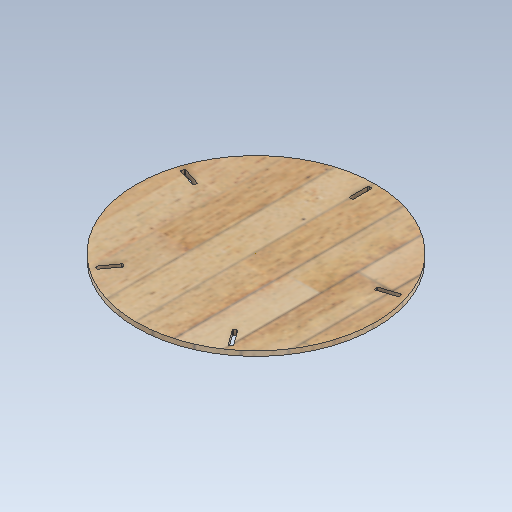
# Autodesk Inventor part: fINAL Roof - G
Saved by Autodesk Inventor 2020 (Build 240168000, 168)
## iProperties
Created: 2020-03-07
Part Number: fINAL Roof - G
Material: Wood (Maple)
Document SubType Name: Sheet Metal
Designer: Daniel Wikman
Density: 0.67 g/cm^3
Sheet Metal Rule: Default_mm
Appearance: Natural Maple - Glossy Dark Tint
Author: Daniel Wikman
Autodesk Inventor part; units mm, degrees
ref_plane "YZ Plane" through (0, 0, 0) normal (1, 0, 0) x (0, 1, 0)
ref_plane "XZ Plane" through (0, 0, 0) normal (0, 1, 0) x (-1, 0, 0)
ref_plane "XY Plane" through (0, 0, 0) normal (0, 0, 1) x (1, 0, 0)
sketch "Sketch1" plane through (0, 0, 0) normal (0, 1, 0) x (-1, 0, 0)
  circle A0 centre (0, 0) radius 200
  dimension "d0" = 400
  constraints: 1 centre point, 1 coincident
  measures "d0" diameter of A0
extrude "Extrusion1" add sketch "Sketch1" along normal blind 8
sketch "Sketch2" plane through (0, 8, 0) normal (0, 1, 0) x (1, 0, 0)
  line L0 (-1.9167, 191.4) -> (1.9167, 191.4)
  line L1 (3.25, 190.0667) -> (3.25, 160.0667)
  line L2 (1.9167, 158.7333) -> (-1.9167, 158.7333)
  line L3 (-3.25, 160.0667) -> (-3.25, 190.0667)
  circle A0 centre (0, 0) radius 200 projected
  arc A1 (-1.9167, 191.4) -> (-3.25, 190.0667) centre (-1.9167, 190.0667) ccw
  arc A2 (3.25, 190.0667) -> (1.9167, 191.4) centre (1.9167, 190.0667) ccw
  arc A3 (1.9167, 158.7333) -> (3.25, 160.0667) centre (1.9167, 160.0667) ccw
  arc A4 (-3.25, 160.0667) -> (-1.9167, 158.7333) centre (-1.9167, 160.0667) ccw
  line L4 (114.1741, -153.6311) -> (111.0728, -155.8843)
  line L5 (109.2104, -155.5893) -> (91.5769, -131.3188)
  line L6 (91.8718, -129.4564) -> (94.9731, -127.2032)
  line L7 (96.8355, -127.4982) -> (114.469, -151.7687)
  arc A5 (114.1741, -153.6311) -> (114.469, -151.7687) centre (113.3904, -152.5524) ccw
  arc A6 (109.2104, -155.5893) -> (111.0728, -155.8843) centre (110.2891, -154.8056) ccw
  arc A7 (91.8718, -129.4564) -> (91.5769, -131.3188) centre (92.6556, -130.5351) ccw
  arc A8 (96.8355, -127.4982) -> (94.9731, -127.2032) centre (95.7568, -128.2819) ccw
  line L8 (181.3689, 61.1875) -> (182.5534, 57.5417)
  line L9 (181.6974, 55.8616) -> (153.1657, 46.5911)
  line L10 (151.4856, 47.4472) -> (150.301, 51.0929)
  line L11 (151.1571, 52.773) -> (179.6888, 62.0435)
  arc A9 (181.3689, 61.1875) -> (179.6888, 62.0435) centre (180.1008, 60.7754) ccw
  arc A10 (181.6974, 55.8616) -> (182.5534, 57.5417) centre (181.2854, 57.1297) ccw
  arc A11 (151.4856, 47.4472) -> (153.1657, 46.5911) centre (152.7537, 47.8592) ccw
  arc A12 (151.1571, 52.773) -> (150.301, 51.0929) centre (151.5691, 51.5049) ccw
  line L12 (-114.1741, -153.6311) -> (-111.0728, -155.8843)
  line L13 (-109.2104, -155.5893) -> (-91.5769, -131.3188)
  line L14 (-91.8718, -129.4564) -> (-94.9731, -127.2032)
  line L15 (-96.8355, -127.4982) -> (-114.469, -151.7687)
  arc A13 (-114.469, -151.7687) -> (-114.1741, -153.6311) centre (-113.3904, -152.5524) ccw
  arc A14 (-111.0728, -155.8843) -> (-109.2104, -155.5893) centre (-110.2891, -154.8056) ccw
  arc A15 (-91.5769, -131.3188) -> (-91.8718, -129.4564) centre (-92.6556, -130.5351) ccw
  arc A16 (-94.9731, -127.2032) -> (-96.8355, -127.4982) centre (-95.7568, -128.2819) ccw
  line L16 (-181.3689, 61.1875) -> (-182.5534, 57.5417)
  line L17 (-181.6974, 55.8616) -> (-153.1657, 46.5911)
  line L18 (-151.4856, 47.4472) -> (-150.301, 51.0929)
  line L19 (-151.1571, 52.773) -> (-179.6888, 62.0435)
  arc A17 (-179.6888, 62.0435) -> (-181.3689, 61.1875) centre (-180.1008, 60.7754) ccw
  arc A18 (-182.5534, 57.5417) -> (-181.6974, 55.8616) centre (-181.2854, 57.1297) ccw
  arc A19 (-153.1657, 46.5911) -> (-151.4856, 47.4472) centre (-152.7537, 47.8592) ccw
  arc A20 (-150.301, 51.0929) -> (-151.1571, 52.773) centre (-151.5691, 51.5049) ccw
  dimension "d3" = 191.4
  dimension "d4" = 6.5
  dimension "d6" = 1.3333
  dimension "d7" = 30
  constraints: 40 end point, 40 point on circle, 20 centre point, 8 tangent, 3 equal radius, 2 parallel, 1 horizontal, 1 perpendicular
  measures "d3" distance from line of A0.centre L0
  measures "d4" distance between parallel lines of L3 L1
  measures "d6" radius of A1
  measures "d7" distance of L1.start L1.end
extrude "Extrusion2" cut sketch "Sketch2" against normal through all contours L0 A2 L1 A3 L2 A4 L3 A1 | L4 A6 L5 A7 L6 A8 L7 A5 | L8 A10 L9 A11 L10 A12 L11 A9 | A13 L15 A16 L14 A15 L13 A14 L12 | A17 L19 A20 L18 A19 L17 A18 L16
equation "\"BendRadius\" = Thickness"
equation "\"BendReliefWidth\" = Thickness"
equation "\"BendReliefDepth\" = 0.5 * Thickness"
equation "\"CornerReliefSize\" = 4 * Thickness"
equation "\"MinimumRemnant\" = 2 * Thickness"
equation "\"TransitionRadius\" = BendRadius"
equation "\"JacobiRadiusSize\" = BendRadius"
equation "\"GapSize\" = Thickness"
equation "\"Thickness\" = 0.5"
body "Solid1"
